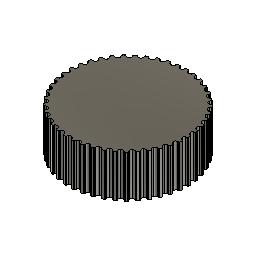
gear_45z (Autodesk Fusion 360 design; units mm, degrees)
Autodesk Fusion 360 part; units mm, degrees
sketch "Sketch1" plane through (0, 0, 0) normal (0, 0, 1) x (1, 0, 0) in component "gt2 pulley"
  circle A0 centre (0, 0) radius 14.3239 construction
  circle A1 centre (0, 0) radius 13.3199 construction
  line L0 (0, 0) -> (0, 14.3239) construction
  line L1 (0, 0) -> (0.9992, 14.2891) construction
  line L2 (0, 0) -> (1.4078, 14.2546) construction
  circle A2 centre (0, 0) radius 14.0699 construction
  arc A3 (0.3855, 13.9289) -> (0.4503, 13.6408) centre (1.3828, 14.0018) ccw
  circle A4 centre (0, 0) radius 13.9199 construction
  arc A5 (0.2384, 14.0679) -> (0, 14.0699) centre (0, 0) ccw
  arc A6 (0.3855, 13.9289) -> (0.2384, 14.0679) centre (0.2359, 13.9179) ccw
  arc A7 (0.4503, 13.6408) -> (0.9292, 13.2875) centre (0.9679, 13.8411) ccw
  arc A8 (0, 14.0699) -> (-0.2384, 14.0679) centre (0, 0) ccw
  arc A9 (-0.2384, 14.0679) -> (-0.3855, 13.9289) centre (-0.2359, 13.9179) ccw
  arc A10 (-0.4503, 13.6408) -> (-0.3855, 13.9289) centre (-1.3828, 14.0018) ccw
  arc A11 (-0.9292, 13.2875) -> (-0.4503, 13.6408) centre (-0.9679, 13.8411) ccw
  arc A12 (0.9292, 13.2875) -> (-0.9292, 13.2875) centre (0, 0) ccw
  point P0 (1.3828, 14.0018)
  point P1 (0, 14.0699)
  dimension "d18" = 28.6479
  dimension "d19" = 4
  dimension "d22" = 1.004
  dimension "d24" = 0.75
  dimension "d26" = 1
  dimension "d27" = 0.15
  dimension "d28" = 0.15
  dimension "d47" = 0.555
  dimension "d52" = 3.812
  constraint coincident A0.centre A1.centre
  constraint coincident A0 L0.end
  constraint vertical L0
  constraint coincident A0 L1.end
  constraint coincident A0 L2.end
  constraint concentric A1 A2
  constraint coincident A1 A7.end
  constraint coincident L1 A7.end
  constraint coincident A2 P0
  constraint coincident L2 P0
  constraint coincident P0 A3.centre
  constraint coincident A2 P1
  constraint coincident L0 P1
  constraint concentric A2 A4
  constraint coincident P1 A5.end
  constraint coincident A4 A6.centre
  constraint coincident A3.start A6.start
  constraint tangent A3 A6
  constraint tangent A3 A7
  constraint symmetric L0 A7.end A11.start
  constraint symmetric L0 A3.start A9.end
  constraint symmetric L0 A3.end A10.start
  constraint symmetric L0 A3 A10
  constraint symmetric L0 A5.start A8.end
  constraint symmetric L0 P1 A5.end
  constraint symmetric L0 A5 A8
  constraint symmetric L0 A6 A9
  constraint symmetric L0 A7 A11
  constraint coincident A1 A11.start
  constraint tangent A1 A7
  constraint coincident L1 A7.centre
  measures "d18" diameter of A0
  measures "d19" angle of L0 L1
  measures "d22" distance of A0 A1
  measures "d24" distance of A1 A2
  measures "d26" radius of A3
  measures "d27" distance of A2 A4
  measures "d28" radius of A6
  measures "d47" radius of A7
extrude "Extrude1" add sketch "Sketch1" along normal blind 10 makes body 1
pattern_circular "C-Pattern1" count 45 over 360 about axis through (0, 0, 1.75) along (0, 0, 1) of bodies 1 makes body 2 at (-1.1352, 13.2715, 3.3333) makes body 3 at (-2.9712, 12.9843, 3.3333) makes body 4 at (-4.7493, 12.4445, 3.3333) makes body 5 at (-6.435, 11.6624, 3.3333) makes body 6 at (-9.1031, 9.724, 6.6667) makes body 7 at (-9.9675, 8.8357, 6.6667) makes body 8 at (-11.4307, 6.8381, 6.6667) makes body 9 at (-12.2711, 5.1807, 6.6667) makes body 10 at (-12.6996, 4.0177, 6.6667) makes body 11 at (-13.1351, 2.2112, 6.6667) makes body 12 at (-13.267, 1.1866, 3.3333) makes body 13 at (-13.1519, -2.1092, 6.6667) makes body 14 at (-12.7303, -3.9191, 6.6667) makes body 15 at (-12.061, -5.6527, 6.6667) makes body 16 at (-11.8799, -6.0241, 3.3333) makes body 17 at (-10.0357, -8.7582, 6.6667) makes body 18 at (-9.1782, -9.6531, 6.6667) makes body 19 at (-7.2329, -11.1851, 6.6667) makes body 20 at (-6.8824, -11.4041, 3.3333) makes body 21 at (-3.8697, -12.7455, 6.6667) makes body 22 at (-3.4724, -12.8594, 3.3333) makes body 23 at (-0.8261, -13.2943, 6.6667) makes body 24 at (0.2066, -13.3183, 3.3333) makes body 25 at (3.4724, -12.8594, 6.6667) makes body 26 at (4.6526, -12.4809, 6.6667) makes body 27 at (6.8824, -11.4041, 6.6667) makes body 28 at (7.9126, -10.715, 6.6667) makes body 29 at (9.7592, -9.0653, 6.6667) makes body 30 at (10.5596, -8.1189, 6.6667) makes body 31 at (11.5867, -6.5703, 6.6667) makes body 32 at (12.061, -5.6527, 3.3333) makes body 33 at (13.0801, -2.5162, 6.6667) makes body 34 at (13.2574, -1.2895, 6.6667) makes body 35 at (13.3174, -0.2583, 3.3333) makes body 36 at (13.2238, 1.5977, 3.3333) makes body 37 at (12.8727, 3.4225, 3.3333) makes body 38 at (12.2711, 5.1807, 3.3333) makes body 39 at (10.6222, 8.0368, 6.6667) makes body 40 at (10.3678, 8.3624, 3.3333) makes body 41 at (7.9955, 10.6533, 6.6667) makes body 42 at (6.9707, 11.3504, 6.6667) makes body 43 at (5.3232, 12.21, 6.6667) makes body 44 at (2.9712, 12.9843, 6.6667) makes body 45 at (1.7514, 13.2043, 6.6667)
sketch "Sketch2" plane through (0, 0, 10) normal (0, 0, 1) x (-1, 0, 0)
  arc A0 (-9.2486, -10.4223) -> (-9.2253, -10.6234) centre (-9.127, -10.5101) ccw
  arc A1 (-9.2253, -10.6234) -> (-8.8601, -10.9299) centre (0, 0) ccw
  arc A2 (-8.8601, -10.9299) -> (-8.658, -10.9179) centre (-8.7656, -10.8134) ccw
  arc A3 (-8.4231, -10.7389) -> (-8.658, -10.9179) centre (-7.9409, -11.6149) ccw
  arc A4 (-7.8293, -10.7761) -> (-8.4231, -10.7389) centre (-8.1555, -11.2251) ccw
  arc A5 (-9.2528, -9.5816) -> (-7.8293, -10.7761) centre (0, 0) ccw
  arc A6 (-9.1131, -10.16) -> (-9.2528, -9.5816) centre (-9.6383, -9.9808) ccw
  arc A7 (-9.2486, -10.4223) -> (-9.1131, -10.16) centre (-10.0595, -9.8371) ccw
  circle A8 centre (0, 0) radius 13.3199
  constraint concentric A1 A8
extrude "Extrude2" add sketch "Sketch2" against normal blind 10 contours A5 A8 bodies 1 2 3 4 5 6 7 8 9 10 11 12 13 14 15 16 17 18 19 20 21 22 23 24 25 26 27 28 29 30 31 32 33 34 35 36 37 38 39 40 41 42 43 44 45
extrude "Extrude4" [suppressed] in component "gt2 pulley"
pattern_circular "C-Pattern7" [suppressed] in component "gt2 pulley"
extrude "Extrude3" [suppressed] in component "gt2 pulley"
pattern_circular "C-Pattern6" [suppressed] in component "gt2 pulley"
extrude "Extrude2'" [suppressed] in component "gt2 pulley"
pattern_circular "C-Pattern5" [suppressed] in component "gt2 pulley"
extrude "Extrude1'" [suppressed] in component "gt2 pulley"
pattern_circular "C-Pattern4" [suppressed] in component "gt2 pulley"
pattern_circular "C-Pattern3" [suppressed] in component "gt2 pulley"
pattern_circular "C-Pattern2" [suppressed] in component "gt2 pulley"
pattern_circular "C-Pattern1'" [suppressed] in component "gt2 pulley"
copy_body "Body->Comp1" [suppressed] in component "Component"
copy_body "Body->Comp2" [suppressed] in component "Component'"
copy_body "Body->Comp3" [suppressed] in component "Component''"
copy_body "Body->Comp4" [suppressed] in component "Component'''"
copy_body "Body->Comp5" [suppressed] in component "Component''''"
copy_body "Body->Comp6" [suppressed] in component "Component'''''"
copy_body "Body->Comp7" [suppressed] in component "Component''''''"
copy_body "Body->Comp8" [suppressed] in component "Component'''''''"
copy_body "Body->Comp9" [suppressed] in component "Component''''''''"
copy_body "Body->Comp10" [suppressed] in component "Component'''''''''"
copy_body "Body->Comp11" [suppressed] in component "Component''''''''''"
copy_body "Body->Comp12" [suppressed] in component "Component'''''''''''"
copy_body "Body->Comp13" [suppressed] in component "Component''''''''''''"
copy_body "Body->Comp14" [suppressed] in component "Component'''''''''''''"
copy_body "Body->Comp15" [suppressed] in component "Component''''''''''''''"
copy_body "Body->Comp16" [suppressed] in component "Component'''''''''''''''"
copy_body "Body->Comp17" [suppressed] in component "Component''''''''''''''''"
copy_body "Body->Comp18" [suppressed] in component "Component'''''''''''''''''"
copy_body "Body->Comp19" [suppressed] in component "Component''''''''''''''''''"
copy_body "Body->Comp20" [suppressed] in component "Component'''''''''''''''''''"
component "gt2 pulley" placed x (1, 0, 0) y (0, 1, 0) z (0, 0, 1) at (0, 0, 0)
equation "NumTeeth = 45" comment "min 20"
equation "ToothPitch = 2 mm"
equation "PullyDia = NumTeeth * ToothPitch / PI"
equation "ToothAng = ( ( 360 / NumTeeth ) * 1 deg )"
equation "TransOffsetAngle = ToothAng * 0.2"
equation "Sholulder_Radius = 0.15 mm"
equation "Root_Radius = 0.555 mm"
equation "TransRadius = 1 mm"
equation "ToolHeight = 0.75 mm"
equation "PLD = 0.254 mm"
equation "d18 = PullyDia"
equation "d19 = ToothAng / 2"
equation "d22 = PLD + ToolHeight"
equation "d24 = ToolHeight"
equation "d26 = TransRadius"
equation "d27 = Sholulder_Radius"
equation "d31 = NumTeeth"
equation "d33 = NumTeeth"
equation "d35 = NumTeeth"
equation "d37 = NumTeeth"
equation "d41 = NumTeeth"
equation "d45 = NumTeeth"
equation "d47 = Root_Radius"
equation "d50 = NumTeeth"
